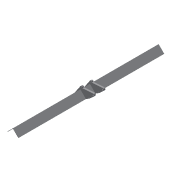
# Autodesk Inventor part: Barra freno
Saved by Autodesk Inventor 2019 (Build 230136000, 136)
## iProperties
Created: 2020-02-07
Part Number: Barra freno
Material: Generic
Document SubType Name: Modeling
Designer: Juan Carlos Botero
Density: 1 g/cm^3
Appearance: Default
Author: Juan Carlos Botero
Autodesk Inventor part; units mm, degrees
ref_plane "YZ Plane" through (0, 0, 0) normal (1, 0, 0) x (0, 1, 0)
ref_plane "XZ Plane" through (0, 0, 0) normal (0, 1, 0) x (-1, 0, 0)
ref_plane "XY Plane" through (0, 0, 0) normal (0, 0, 1) x (1, 0, 0)
sketch "Sketch1" plane through (0, 0, 0) normal (0, 0, 1) x (1, 0, 0)
  line L0 (0, 0) -> (42.4264, -42.4264)
  line L1 (-42.4264, -42.4264) -> (0, 0)
  line L2 (42.4264, -42.4264) -> (40.6586, -44.1942)
  line L3 (40.6586, -44.1942) -> (0, -3.5355)
  line L4 (0, -3.5355) -> (-40.6586, -44.1942)
  line L5 (-40.6586, -44.1942) -> (-42.4264, -42.4264)
  dimension "d0" = 2.5
  dimension "d1" = 60
  constraints: 12 end point, 7 perpendicular, 1 vertical alignment
  measures "d0" distance of L0.end L2.end
  measures "d1" distance of L0.start L0.end
extrude "Extrusion1" add sketch "Sketch1" along normal mid plane 1100
sketch "Sketch2" plane through (0, 0, 0) normal (0, 0, 1) x (1, 0, 0)
  circle A0 centre (139.8689, 6.067) radius 5
  circle A1 centre (68.2145, -29.7861) radius 3
  circle A2 centre (68.272, 15.9062) radius 3
  line L0 (42.4264, -42.4264) -> (0, 0) projected
  circle A3 centre (139.8689, 6.067) radius 10
  line L1 (0, 0) -> (-42.4264, -42.4264) projected
  arc A4 (76.2705, 16.0588) -> (65.5794, 23.4394) centre (68.272, 15.9062) ccw
  circle A5 centre (68.2145, -29.7861) radius 7.5
  line L2 (42.4264, -42.4264) -> (69.6422, -37.1489)
  line L3 (71.3596, -36.5947) -> (144.0624, -3.0112)
  line L4 (76.2705, 16.0588) -> (139.8676, 16.067)
  line L5 (0, 0) -> (65.5794, 23.4394)
  dimension "d4" = 10
  dimension "d5" = 6
  dimension "d6" = 6
  dimension "d7" = 20
  dimension "d9" = 8
  dimension "d10" = 15
  constraints: 8 end point, 6 centre point, 6 point on circle, 5 tangent, 2 coincident, 1 concentric
  measures "d4" diameter of A0
  measures "d5" diameter of A1
  measures "d6" diameter of A2
  measures "d7" diameter of A3
  measures "d9" radius of A4
  measures "d10" diameter of A5
extrude "Extrusion2" add sketch "Sketch2" along normal mid plane 6 separate body
body "Solid1"
body "Solid2"
